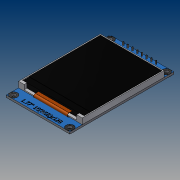
# Autodesk Inventor part: 1e77-TFT-160x128
Saved by Autodesk Inventor 2022.3 (Build 263350000, 350)
## iProperties
Created: 2022-05-13
Part Number: 1e77-TFT-160x128
Material: Generico
Document SubType Name: Modeling
Designer: Bat
Density: 1 g/cm^3
Appearance: Default
Peso: =<MASS>
Author: Bat
Autodesk Inventor part; units mm, degrees
(part 1 of 2)
ref_plane "YZ Plane" through (0, 0, 0) normal (1, 0, 0) x (0, 1, 0)
ref_plane "XZ Plane" through (0, 0, 0) normal (0, 1, 0) x (-1, 0, 0)
ref_plane "XY Plane" through (0, 0, 0) normal (0, 0, 1) x (1, 0, 0)
sketch "Schizzo1" plane through (0, 0, 0) normal (0, 0, 1) x (1, 0, 0)
  line L0 (-17, 27.75) -> (17, 27.75)
  line L1 (17, 27.75) -> (17, -27.75)
  line L2 (17, -27.75) -> (-17, -27.75)
  line L3 (-17, -27.75) -> (-17, 27.75)
  line L4 (-17, 27.75) -> (17, -27.75) construction
  line L5 (17, 27.75) -> (-17, -27.75) construction
  point P0 (0, 0)
  dimension "d0" = 34
  dimension "d1" = 55.5
  constraints: 12 end point, 2 midpoint, 2 parallel, 1 horizontal, 1 perpendicular
  measures "d0" distance of L1.end L2.end
  measures "d1" distance of L0.end L1.end
extrude "Estrusione1" add sketch "Schizzo1" along normal mid plane 1.1
sketch "Schizzo2" plane through (0, 0, 0.55) normal (0, 0, 1) x (1, 0, 0)
  line L0 (-15, -25.75) -> (15, -25.75)
  line L1 (15, -25.75) -> (15, 25.75)
  line L2 (15, 25.75) -> (-15, 25.75)
  line L3 (-15, 25.75) -> (-15, -25.75)
  line L4 (-15, -25.75) -> (15, 25.75) construction
  line L5 (15, -25.75) -> (-15, 25.75) construction
  point P0 (0, 0)
  dimension "d4" = 30
  dimension "d5" = 51.5
  constraints: 12 end point, 2 midpoint, 2 parallel, 1 horizontal, 1 perpendicular
  measures "d4" distance of L1.end L2.end
  measures "d5" distance of L0.end L1.end
hole "Foro1" at (-15, 25.75, 0.55) at (15, 25.75, 0.55) at (-15, -25.75, 0.55) at (15, -25.75, 0.55) direction (0, 0, -1) diameter 2.1 end through all
sketch "Schizzo3" plane through (0, 0, 0.55) normal (0, 0, 1) x (1, 0, 0)
  circle A0 centre (-15, 25.75) radius 1.05 projected
  circle A1 centre (-15, 25.75) radius 2
  line L0 (-23.8, 0) -> (23.8, 0) construction
  line L1 (0, 38.85) -> (0, -38.85) construction
  circle A2 centre (15, 25.75) radius 1.05
  circle A3 centre (15, 25.75) radius 2
  circle A4 centre (-15, -25.75) radius 1.05
  circle A5 centre (-15, -25.75) radius 2
  circle A6 centre (15, -25.75) radius 2
  circle A7 centre (15, -25.75) radius 1.05
  point P0 (0, 0)
  dimension "d13" = 4
  constraints: 7 centre point, 6 symmetric about line, 4 coincident, 6 other
  measures "d13" diameter of A1
extrude "Estrusione2" add sketch "Schizzo3" along normal blind 0.05
mirror "Specchio1" about plane through (0, 0, 0) normal (0, 0, 1) of "Estrusione2"
sketch "Schizzo4" plane through (0, 0, 0.55) normal (0, 0, 1) x (1, 0, 0)
  line L0 (-9, 12.35) -> (-3.8, 12.35)
  line L1 (-3.8, 12.35) -> (-3.8, 9.55)
  line L2 (-3.8, 9.55) -> (-9, 9.55)
  line L3 (-9, 9.55) -> (-9, 12.35)
  line L4 (-9, 12.35) -> (-3.8, 9.55) construction
  line L5 (-3.8, 12.35) -> (-9, 9.55) construction
  line L6 (15, 27.75) -> (-15, 27.75) construction
  line L7 (-17, 25.75) -> (-17, -25.75) construction
  line L8 (-9, 9.15) -> (-3.8, 9.15)
  line L9 (-3.8, 9.15) -> (-3.8, 6.35)
  line L10 (-3.8, 6.35) -> (-9, 6.35)
  line L11 (-9, 6.35) -> (-9, 9.15)
  line L12 (-9, 9.15) -> (-3.8, 6.35) construction
  line L13 (-3.8, 9.15) -> (-9, 6.35) construction
  line L14 (-9, 5.95) -> (-3.8, 5.95)
  line L15 (-3.8, 5.95) -> (-3.8, 3.15)
  line L16 (-3.8, 3.15) -> (-9, 3.15)
  line L17 (-9, 3.15) -> (-9, 5.95)
  line L18 (-9, 5.95) -> (-3.8, 3.15) construction
  line L19 (-3.8, 5.95) -> (-9, 3.15) construction
  line L20 (-2, 7.95) -> (3.2, 7.95)
  line L21 (3.2, 7.95) -> (3.2, 10.75)
  line L22 (3.2, 10.75) -> (-2, 10.75)
  line L23 (-2, 10.75) -> (-2, 7.95)
  line L24 (-2, 7.95) -> (3.2, 10.75) construction
  line L25 (3.2, 7.95) -> (-2, 10.75) construction
  line L26 (-2, 7.55) -> (3.2, 7.55)
  line L27 (3.2, 7.55) -> (3.2, 4.75)
  line L28 (3.2, 4.75) -> (-2, 4.75)
  line L29 (-2, 4.75) -> (-2, 7.55)
  line L30 (-2, 7.55) -> (3.2, 4.75) construction
  line L31 (3.2, 7.55) -> (-2, 4.75) construction
  line L32 (6.3, 13.25) -> (11.5, 13.25)
  line L33 (11.5, 13.25) -> (11.5, 10.45)
  line L34 (11.5, 10.45) -> (6.3, 10.45)
  line L35 (6.3, 10.45) -> (6.3, 13.25)
  line L36 (6.3, 13.25) -> (11.5, 10.45) construction
  line L37 (11.5, 13.25) -> (6.3, 10.45) construction
  line L38 (17, -25.75) -> (17, 25.75) construction
  line L39 (-11.7056, 11.7024) -> (-9.3, 11.7024) construction
  line L40 (-9.3, 11.7024) -> (-9.3, 10.1976) construction
  line L41 (-9.3, 10.1976) -> (-11.7056, 10.1976) construction
  line L42 (-11.7056, 10.1976) -> (-11.7056, 11.7024) construction
  line L43 (-11.7056, 8.5024) -> (-9.3, 8.5024) construction
  line L44 (-9.3, 8.5024) -> (-9.3, 6.9976) construction
  line L45 (-9.3, 6.9976) -> (-11.7056, 6.9976) construction
  line L46 (-11.7056, 6.9976) -> (-11.7056, 8.5024) construction
  line L47 (-11.7056, 5.3024) -> (-9.3, 5.3024) construction
  line L48 (-9.3, 5.3024) -> (-9.3, 3.7976) construction
  line L49 (-9.3, 3.7976) -> (-11.7056, 3.7976) construction
  line L50 (-11.7056, 3.7976) -> (-11.7056, 5.3024) construction
  line L51 (3.5, 10.1024) -> (5.9056, 10.1024) construction
  line L52 (5.9056, 10.1024) -> (5.9056, 8.5976) construction
  line L53 (5.9056, 8.5976) -> (3.5, 8.5976) construction
  line L54 (3.5, 8.5976) -> (3.5, 10.1024) construction
  line L55 (3.5, 5.3976) -> (3.5, 6.9024) construction
  line L56 (3.5, 6.9024) -> (5.9056, 6.9024) construction
  line L57 (5.9056, 6.9024) -> (5.9056, 5.3976) construction
  line L58 (5.9056, 5.3976) -> (3.5, 5.3976) construction
  line L59 (11.8, 11.0976) -> (11.8, 12.6024) construction
  line L60 (11.8, 12.6024) -> (14.2056, 12.6024) construction
  line L61 (14.2056, 12.6024) -> (14.2056, 11.0976) construction
  line L62 (14.2056, 11.0976) -> (11.8, 11.0976) construction
  line L63 (6.3, 16.25) -> (9.8, 16.25)
  line L64 (9.8, 16.25) -> (9.8, 14.25)
  line L65 (9.8, 14.25) -> (6.3, 14.25)
  line L66 (6.3, 14.25) -> (6.3, 16.25)
  line L67 (6.3, 16.25) -> (9.8, 14.25) construction
  line L68 (9.8, 16.25) -> (6.3, 14.25) construction
  line L69 (10.1951, 16.4758) -> (10.1951, 17.9806) construction
  line L70 (10.1951, 17.9806) -> (12.6007, 17.9806) construction
  line L71 (12.6007, 17.9806) -> (12.6007, 16.4758) construction
  line L72 (12.6007, 16.4758) -> (10.1951, 16.4758) construction
  line L73 (-1.2, 15.8215) -> (-0.2, 15.8215)
  line L74 (-0.2, 15.8215) -> (-0.2, 13.3215)
  line L75 (-0.2, 13.3215) -> (-1.2, 13.3215)
  line L76 (-1.2, 13.3215) -> (-1.2, 15.8215)
  line L77 (-1.2, 15.8215) -> (-0.2, 13.3215) construction
  line L78 (-0.2, 15.8215) -> (-1.2, 13.3215) construction
  line L79 (0.1593, 15.9667) -> (0.1593, 17.4716) construction
  line L80 (0.1593, 17.4716) -> (2.5649, 17.4716) construction
  line L81 (2.5649, 17.4716) -> (2.5649, 15.9667) construction
  line L82 (2.5649, 15.9667) -> (0.1593, 15.9667) construction
  line L83 (-13.9282, 19.8471) -> (-2.7925, 19.8471) construction
  line L84 (-2.7925, 19.8471) -> (-2.7925, 18.2669) construction
  line L85 (-2.7925, 18.2669) -> (-13.9282, 18.2669) construction
  line L86 (-13.9282, 18.2669) -> (-13.9282, 19.8471) construction
  line L87 (-3.95, 12.2) -> (-8.85, 12.2)
  line L88 (-8.85, 12.2) -> (-8.85, 9.7)
  line L89 (-8.85, 9.7) -> (-3.95, 9.7)
  line L90 (-3.95, 9.7) -> (-3.95, 12.2)
  line L91 (-3.95, 9) -> (-8.85, 9)
  line L92 (-8.85, 9) -> (-8.85, 6.5)
  line L93 (-8.85, 6.5) -> (-3.95, 6.5)
  line L94 (-3.95, 6.5) -> (-3.95, 9)
  line L95 (-3.95, 5.8) -> (-8.85, 5.8)
  line L96 (-8.85, 5.8) -> (-8.85, 3.3)
  line L97 (-8.85, 3.3) -> (-3.95, 3.3)
  line L98 (-3.95, 3.3) -> (-3.95, 5.8)
  line L99 (-1.85, 10.6) -> (3.05, 10.6)
  line L100 (3.05, 10.6) -> (3.05, 8.1)
  line L101 (3.05, 8.1) -> (-1.85, 8.1)
  line L102 (-1.85, 8.1) -> (-1.85, 10.6)
  line L103 (3.05, 7.4) -> (-1.85, 7.4)
  line L104 (-1.85, 7.4) -> (-1.85, 4.9)
  line L105 (-1.85, 4.9) -> (3.05, 4.9)
  line L106 (3.05, 4.9) -> (3.05, 7.4)
  line L107 (11.35, 13.1) -> (6.45, 13.1)
  line L108 (6.45, 13.1) -> (6.45, 10.6)
  line L109 (6.45, 10.6) -> (11.35, 10.6)
  line L110 (11.35, 10.6) -> (11.35, 13.1)
  line L111 (9.65, 16.1) -> (6.45, 16.1)
  line L112 (6.45, 16.1) -> (6.45, 14.4)
  line L113 (6.45, 14.4) -> (9.65, 14.4)
  line L114 (9.65, 14.4) -> (9.65, 16.1)
  line L115 (-0.35, 15.6715) -> (-1.05, 15.6715)
  line L116 (-1.05, 15.6715) -> (-1.05, 13.4715)
  line L117 (-1.05, 13.4715) -> (-0.35, 13.4715)
  line L118 (-0.35, 13.4715) -> (-0.35, 15.6715)
  line L119 (-10.3928, 10.1976) -> (-10.6517, 10.1976)
  line L120 (-10.6517, 10.1976) -> (-11.1258, 10.7944)
  line L121 (-11.1258, 10.7944) -> (-11.3543, 10.7944)
  line L122 (-11.3543, 10.7944) -> (-11.3543, 10.1976)
  line L123 (-11.3543, 10.1976) -> (-11.5536, 10.1976)
  line L124 (-11.5536, 10.1976) -> (-11.5536, 11.6976)
  line L125 (-11.5536, 11.6976) -> (-11.1671, 11.6976)
  spline S0 degree 2 poles (-11.1671, 11.6976) (-11.0382, 11.6976) (-10.8644, 11.6696) (-10.7854, 11.6186) knots 0 0 0 1 2 2 2
  spline S1 degree 2 poles (-10.7854, 11.6186) (-10.7064, 11.5675) (-10.6152, 11.4083) (-10.6152, 11.2904) knots 0 0 0 1 2 2 2
  spline S2 degree 2 poles (-10.6152, 11.2904) (-10.6152, 11.1263) (-10.783, 10.9038) (-10.9264, 10.8503) knots 0 0 0 1 2 2 2
  line L126 (-10.9264, 10.8503) -> (-10.3928, 10.1976)
  spline S3 degree 2 poles (-10.8231, 11.2746) (-10.8231, 11.3402) (-10.8693, 11.4411) (-10.9179, 11.4739) knots 0 0 0 1 2 2 2
  spline S4 degree 2 poles (-10.9179, 11.4739) (-10.9605, 11.5019) (-11.0735, 11.525) (-11.1562, 11.525) knots 0 0 0 1 2 2 2
  line L127 (-11.1562, 11.525) -> (-11.3543, 11.525)
  line L128 (-11.3543, 11.525) -> (-11.3543, 10.9609)
  line L129 (-11.3543, 10.9609) -> (-11.1793, 10.9609)
  spline S5 degree 2 poles (-11.1793, 10.9609) (-11.0929, 10.9609) (-10.9556, 10.9913) (-10.9082, 11.0387) knots 0 0 0 1 2 2 2
  spline S6 degree 2 poles (-10.9082, 11.0387) (-10.8644, 11.0801) (-10.8231, 11.1968) (-10.8231, 11.2746) knots 0 0 0 1 2 2 2
  line L130 (-9.4665, 10.1976) -> (-10.1983, 10.1976)
  line L131 (-10.1983, 10.1976) -> (-10.1983, 10.3507)
  line L132 (-10.1983, 10.3507) -> (-9.926, 10.3507)
  line L133 (-9.926, 10.3507) -> (-9.926, 11.356)
  line L134 (-9.926, 11.356) -> (-10.1983, 11.356)
  line L135 (-10.1983, 11.356) -> (-10.1983, 11.4934)
  spline S7 degree 2 poles (-10.1983, 11.4934) (-10.0439, 11.4934) (-9.8981, 11.5809) (-9.8883, 11.7024) knots 0 0 0 1 2 2 2
  line L136 (-9.8883, 11.7024) -> (-9.7327, 11.7024)
  line L137 (-9.7327, 11.7024) -> (-9.7327, 10.3507)
  line L138 (-9.7327, 10.3507) -> (-9.4665, 10.3507)
  line L139 (-9.4665, 10.3507) -> (-9.4665, 10.1976)
  spline S8 degree 2 poles (0.7, 16.1045) (0.594, 16.1045) (0.4364, 16.16) (0.381, 16.2154) knots 0 0 0 1 2 2 2
  spline S9 degree 2 poles (0.381, 16.2154) (0.3178, 16.2776) (0.2663, 16.4527) (0.2663, 16.581) knots 0 0 0 1 2 2 2
  line L140 (0.2663, 16.581) -> (0.2663, 17.3298)
  line L141 (0.2663, 17.3298) -> (0.4257, 17.3298)
  line L142 (0.4257, 17.3298) -> (0.4257, 16.581)
  spline S10 degree 2 poles (0.4257, 16.581) (0.4257, 16.4974) (0.4471, 16.3846) (0.4773, 16.3389) knots 0 0 0 1 2 2 2
  spline S11 degree 2 poles (0.4773, 16.3389) (0.5094, 16.2903) (0.6202, 16.2407) (0.7, 16.2407) knots 0 0 0 1 2 2 2
  spline S12 degree 2 poles (0.7, 16.2407) (0.7748, 16.2407) (0.8915, 16.2903) (0.9236, 16.3389) knots 0 0 0 1 2 2 2
  spline S13 degree 2 poles (0.9236, 16.3389) (0.9538, 16.3846) (0.9752, 16.4964) (0.9752, 16.5772) knots 0 0 0 1 2 2 2
  line L143 (0.9752, 16.5772) -> (0.9752, 17.3298)
  line L144 (0.9752, 17.3298) -> (1.1346, 17.3298)
  line L145 (1.1346, 17.3298) -> (1.1346, 16.581)
  spline S14 degree 2 poles (1.1346, 16.581) (1.1346, 16.4556) (1.0841, 16.2767) (1.0199, 16.2154) knots 0 0 0 1 2 2 2
  spline S15 degree 2 poles (1.0199, 16.2154) (0.9625, 16.159) (0.8108, 16.1045) (0.7, 16.1045) knots 0 0 0 1 2 2 2
  line L146 (2.0089, 16.1298) -> (1.4235, 16.1298)
  line L147 (1.4235, 16.1298) -> (1.4235, 16.2524)
  line L148 (1.4235, 16.2524) -> (1.6413, 16.2524)
  line L149 (1.6413, 16.2524) -> (1.6413, 17.0566)
  line L150 (1.6413, 17.0566) -> (1.4235, 17.0566)
  line L151 (1.4235, 17.0566) -> (1.4235, 17.1665)
  spline S16 degree 2 poles (1.4235, 17.1665) (1.547, 17.1665) (1.6637, 17.2365) (1.6714, 17.3337) knots 0 0 0 1 2 2 2
  line L152 (1.6714, 17.3337) -> (1.7959, 17.3337)
  line L153 (1.7959, 17.3337) -> (1.7959, 16.2524)
  line L154 (1.7959, 16.2524) -> (2.0089, 16.2524)
  line L155 (2.0089, 16.2524) -> (2.0089, 16.1298)
  line L156 (-12.794, 17.1939) -> (-13.6585, 17.1939)
  line L157 (-13.6585, 17.1939) -> (-13.6585, 17.4533)
  line L158 (-13.6585, 17.4533) -> (-13.3374, 17.4533)
  line L159 (-13.3374, 17.4533) -> (-13.3374, 19.1555)
  line L160 (-13.3374, 19.1555) -> (-13.6585, 19.1555)
  line L161 (-13.6585, 19.1555) -> (-13.6585, 19.3881)
  spline S17 degree 2 poles (-13.6585, 19.3881) (-13.4774, 19.3881) (-13.3045, 19.5363) (-13.2942, 19.7422) knots 0 0 0 1 2 2 2
  line L162 (-13.2942, 19.7422) -> (-13.109, 19.7422)
  line L163 (-13.109, 19.7422) -> (-13.109, 17.4533)
  line L164 (-13.109, 17.4533) -> (-12.794, 17.4533)
  line L165 (-12.794, 17.4533) -> (-12.794, 17.1939)
  line L166 (-12.0839, 17.1939) -> (-12.368, 17.1939)
  line L167 (-12.368, 17.1939) -> (-12.368, 17.6797)
  line L168 (-12.368, 17.6797) -> (-12.0839, 17.6797)
  line L169 (-12.0839, 17.6797) -> (-12.0839, 17.1939)
  line L170 (-10.6122, 19.3531) -> (-11.38, 17.1939)
  line L171 (-11.38, 17.1939) -> (-11.6331, 17.1939)
  line L172 (-11.6331, 17.1939) -> (-10.8221, 19.4355)
  line L173 (-10.8221, 19.4355) -> (-11.7381, 19.4355)
  line L174 (-11.7381, 19.4355) -> (-11.7381, 19.7339)
  line L175 (-11.7381, 19.7339) -> (-10.6122, 19.7339)
  line L176 (-10.6122, 19.7339) -> (-10.6122, 19.3531)
  line L177 (-9.2784, 19.3531) -> (-10.0462, 17.1939)
  line L178 (-10.0462, 17.1939) -> (-10.2993, 17.1939)
  line L179 (-10.2993, 17.1939) -> (-9.4883, 19.4355)
  line L180 (-9.4883, 19.4355) -> (-10.4043, 19.4355)
  line L181 (-10.4043, 19.4355) -> (-10.4043, 19.7339)
  line L182 (-10.4043, 19.7339) -> (-9.2784, 19.7339)
  line L183 (-9.2784, 19.7339) -> (-9.2784, 19.3531)
  line L184 (-8.3439, 19.8471) -> (-8.3954, 18.8591)
  line L185 (-8.3954, 18.8591) -> (-8.5518, 18.8591)
  line L186 (-8.5518, 18.8591) -> (-8.6032, 19.8471)
  line L187 (-8.6032, 19.8471) -> (-8.3439, 19.8471)
  line L188 (-8.7926, 19.8471) -> (-8.8441, 18.8591)
  line L189 (-8.8441, 18.8591) -> (-9.0005, 18.8591)
  line L190 (-9.0005, 18.8591) -> (-9.052, 19.8471)
  line L191 (-9.052, 19.8471) -> (-8.7926, 19.8471)
  line L192 (-6.8495, 17.1939) -> (-6.8495, 19.4334)
  line L193 (-6.8495, 19.4334) -> (-7.4465, 19.4334)
  line L194 (-7.4465, 19.4334) -> (-7.4465, 19.7339)
  line L195 (-7.4465, 19.7339) -> (-6.0159, 19.7339)
  line L196 (-6.0159, 19.7339) -> (-6.0159, 19.4334)
  line L197 (-6.0159, 19.4334) -> (-6.6128, 19.4334)
  line L198 (-6.6128, 19.4334) -> (-6.6128, 17.1939)
  line L199 (-6.6128, 17.1939) -> (-6.8495, 17.1939)
  line L200 (-4.7768, 19.4334) -> (-5.6022, 19.4334)
  line L201 (-5.6022, 19.4334) -> (-5.6022, 18.7171)
  line L202 (-5.6022, 18.7171) -> (-4.8118, 18.7171)
  line L203 (-4.8118, 18.7171) -> (-4.8118, 18.4166)
  line L204 (-4.8118, 18.4166) -> (-5.6022, 18.4166)
  line L205 (-5.6022, 18.4166) -> (-5.6022, 17.1939)
  line L206 (-5.6022, 17.1939) -> (-5.8389, 17.1939)
  line L207 (-5.8389, 17.1939) -> (-5.8389, 19.7339)
  line L208 (-5.8389, 19.7339) -> (-4.7768, 19.7339)
  line L209 (-4.7768, 19.7339) -> (-4.7768, 19.4334)
  line L210 (-4.149, 17.1939) -> (-4.149, 19.4334)
  line L211 (-4.149, 19.4334) -> (-4.7459, 19.4334)
  line L212 (-4.7459, 19.4334) -> (-4.7459, 19.7339)
  line L213 (-4.7459, 19.7339) -> (-3.3154, 19.7339)
  line L214 (-3.3154, 19.7339) -> (-3.3154, 19.4334)
  line L215 (-3.3154, 19.4334) -> (-3.9123, 19.4334)
  line L216 (-3.9123, 19.4334) -> (-3.9123, 17.1939)
  line L217 (-3.9123, 17.1939) -> (-4.149, 17.1939)
  line L218 (-10.3928, 7) -> (-10.6517, 7)
  line L219 (-10.6517, 7) -> (-11.1258, 7.5968)
  line L220 (-11.1258, 7.5968) -> (-11.3543, 7.5968)
  line L221 (-11.3543, 7.5968) -> (-11.3543, 7)
  line L222 (-11.3543, 7) -> (-11.5536, 7)
  line L223 (-11.5536, 7) -> (-11.5536, 8.5)
  line L224 (-11.5536, 8.5) -> (-11.1671, 8.5)
  spline S18 degree 2 poles (-11.1671, 8.5) (-11.0382, 8.5) (-10.8644, 8.472) (-10.7854, 8.421) knots 0 0 0 1 2 2 2
  spline S19 degree 2 poles (-10.7854, 8.421) (-10.7064, 8.3699) (-10.6152, 8.2107) (-10.6152, 8.0928) knots 0 0 0 1 2 2 2
  spline S20 degree 2 poles (-10.6152, 8.0928) (-10.6152, 7.9287) (-10.783, 7.7062) (-10.9264, 7.6528) knots 0 0 0 1 2 2 2
  line L225 (-10.9264, 7.6528) -> (-10.3928, 7)
  spline S21 degree 2 poles (-10.8231, 8.077) (-10.8231, 8.1426) (-10.8693, 8.2435) (-10.9179, 8.2763) knots 0 0 0 1 2 2 2
  spline S22 degree 2 poles (-10.9179, 8.2763) (-10.9605, 8.3043) (-11.0735, 8.3274) (-11.1562, 8.3274) knots 0 0 0 1 2 2 2
  line L226 (-11.1562, 8.3274) -> (-11.3543, 8.3274)
  line L227 (-11.3543, 8.3274) -> (-11.3543, 7.7634)
  line L228 (-11.3543, 7.7634) -> (-11.1793, 7.7634)
  spline S23 degree 2 poles (-11.1793, 7.7634) (-11.0929, 7.7634) (-10.9556, 7.7938) (-10.9082, 7.8412) knots 0 0 0 1 2 2 2
  spline S24 degree 2 poles (-10.9082, 7.8412) (-10.8644, 7.8825) (-10.8231, 7.9992) (-10.8231, 8.077) knots 0 0 0 1 2 2 2
  spline S25 degree 2 poles (-9.9114, 8.3578) (-9.9661, 8.3578) (-10.0743, 8.331) (-10.1266, 8.3104) knots 0 0 0 1 2 2 2
  spline S26 degree 2 poles (-10.1266, 8.3104) (-10.1752, 8.2897) (-10.2469, 8.2459) (-10.2749, 8.2265) knots 0 0 0 1 2 2 2
  line L229 (-10.2749, 8.2265) -> (-10.287, 8.2265)
  line L230 (-10.287, 8.2265) -> (-10.287, 8.4392)
  spline S27 degree 2 poles (-10.287, 8.4392) (-10.2214, 8.4745) (-9.9965, 8.5316) (-9.8956, 8.5316) knots 0 0 0 1 2 2 2
  spline S28 degree 2 poles (-9.8956, 8.5316) (-9.7935, 8.5316) (-9.6416, 8.4903) (-9.5796, 8.4465) knots 0 0 0 1 2 2 2
  spline S29 degree 2 poles (-9.5796, 8.4465) (-9.5139, 8.3991) (-9.4459, 8.2618) (-9.4459, 8.1694) knots 0 0 0 1 2 2 2
  spline S30 degree 2 poles (-9.4459, 8.1694) (-9.4459, 8.0454) (-9.6088, 7.8582) (-9.723, 7.8339) knots 0 0 0 1 2 2 2
  line L231 (-9.723, 7.8339) -> (-9.723, 7.8193)
  spline S31 degree 2 poles (-9.723, 7.8193) (-9.6756, 7.8096) (-9.5674, 7.7658) (-9.5212, 7.722) knots 0 0 0 1 2 2 2
  spline S32 degree 2 poles (-9.5212, 7.722) (-9.475, 7.6795) (-9.4167, 7.5434) (-9.4167, 7.4449) knots 0 0 0 1 2 2 2
  spline S33 degree 2 poles (-9.4167, 7.4449) (-9.4167, 7.344) (-9.486, 7.1726) (-9.5492, 7.107) knots 0 0 0 1 2 2 2
  spline S34 degree 2 poles (-9.5492, 7.107) (-9.6148, 7.0389) (-9.8008, 6.9684) (-9.9187, 6.9684) knots 0 0 0 1 2 2 2
  spline S35 degree 2 poles (-9.9187, 6.9684) (-10.0318, 6.9684) (-10.253, 7.0231) (-10.3284, 7.0608) knots 0 0 0 1 2 2 2
  line L232 (-10.3284, 7.0608) -> (-10.3284, 7.2735)
  line L233 (-10.3284, 7.2735) -> (-10.3138, 7.2735)
  spline S36 degree 2 poles (-10.3138, 7.2735) (-10.2506, 7.2273) (-10.0366, 7.1422) (-9.9309, 7.1422) knots 0 0 0 1 2 2 2
  spline S37 degree 2 poles (-9.9309, 7.1422) (-9.8689, 7.1422) (-9.7449, 7.1811) (-9.7036, 7.2261) knots 0 0 0 1 2 2 2
  spline S38 degree 2 poles (-9.7036, 7.2261) (-9.6635, 7.2711) (-9.6209, 7.378) (-9.6209, 7.4595) knots 0 0 0 1 2 2 2
  spline S39 degree 2 poles (-9.6209, 7.4595) (-9.6209, 7.5409) (-9.6683, 7.6467) (-9.7109, 7.6771) knots 0 0 0 1 2 2 2
  spline S40 degree 2 poles (-9.7109, 7.6771) (-9.7534, 7.7075) (-9.8689, 7.7306) (-9.937, 7.7306) knots 0 0 0 1 2 2 2
  line L234 (-9.937, 7.7306) -> (-10.022, 7.7306)
  line L235 (-10.022, 7.7306) -> (-10.022, 7.8971)
  line L236 (-10.022, 7.8971) -> (-9.9552, 7.8971)
  spline S41 degree 2 poles (-9.9552, 7.8971) (-9.8203, 7.8971) (-9.6501, 8.0259) (-9.6501, 8.1487) knots 0 0 0 1 2 2 2
  spline S42 degree 2 poles (-9.6501, 8.1487) (-9.6501, 8.2058) (-9.6938, 8.2873) (-9.7291, 8.3116) knots 0 0 0 1 2 2 2
  spline S43 degree 2 poles (-9.7291, 8.3116) (-9.7668, 8.3371) (-9.8592, 8.3578) (-9.9114, 8.3578) knots 0 0 0 1 2 2 2
  spline S44 degree 2 poles (-10.9264, 3.7733) (-11.0723, 3.7733) (-11.319, 3.8717) (-11.409, 3.9702) knots 0 0 0 1 2 2 2
  spline S45 degree 2 poles (-11.409, 3.9702) (-11.4989, 4.0674) (-11.5974, 4.3592) (-11.5974, 4.5488) knots 0 0 0 1 2 2 2
  spline S46 degree 2 poles (-11.5974, 4.5488) (-11.5974, 4.7372) (-11.5014, 5.0168) (-11.4102, 5.1201) knots 0 0 0 1 2 2 2
  spline S47 degree 2 poles (-11.4102, 5.1201) (-11.3203, 5.221) (-11.0747, 5.3267) (-10.9228, 5.3267) knots 0 0 0 1 2 2 2
  spline S48 degree 2 poles (-10.9228, 5.3267) (-10.8474, 5.3267) (-10.7149, 5.3049) (-10.659, 5.2878) knots 0 0 0 1 2 2 2
  spline S49 degree 2 poles (-10.659, 5.2878) (-10.6104, 5.272) (-10.5095, 5.2271) (-10.4596, 5.2003) knots 0 0 0 1 2 2 2
  line L237 (-10.4596, 5.2003) -> (-10.4596, 4.9596)
  line L238 (-10.4596, 4.9596) -> (-10.4754, 4.9596)
  spline S50 degree 2 poles (-10.4754, 4.9596) (-10.5022, 4.984) (-10.5848, 5.052) (-10.6444, 5.0848) knots 0 0 0 1 2 2 2
  spline S51 degree 2 poles (-10.6444, 5.0848) (-10.7015, 5.1165) (-10.8365, 5.1566) (-10.924, 5.1566) knots 0 0 0 1 2 2 2
  spline S52 degree 2 poles (-10.924, 5.1566) (-11.02, 5.1566) (-11.1914, 5.0776) (-11.2558, 5.0022) knots 0 0 0 1 2 2 2
  spline S53 degree 2 poles (-11.2558, 5.0022) (-11.319, 4.9256) (-11.3895, 4.6934) (-11.3895, 4.5488) knots 0 0 0 1 2 2 2
  spline S54 degree 2 poles (-11.3895, 4.5488) (-11.3895, 4.3944) (-11.3154, 4.172) (-11.251, 4.0954) knots 0 0 0 1 2 2 2
  spline S55 degree 2 poles (-11.251, 4.0954) (-11.1878, 4.0212) (-11.0188, 3.9459) (-10.924, 3.9459) knots 0 0 0 1 2 2 2
  spline S56 degree 2 poles (-10.924, 3.9459) (-10.8377, 3.9459) (-10.6906, 3.9884) (-10.6335, 4.02) knots 0 0 0 1 2 2 2
  spline S57 degree 2 poles (-10.6335, 4.02) (-10.5788, 4.0516) (-10.4973, 4.1173) (-10.4742, 4.1404) knots 0 0 0 1 2 2 2
  line L239 (-10.4742, 4.1404) -> (-10.4596, 4.1404)
  line L240 (-10.4596, 4.1404) -> (-10.4596, 3.9021)
  spline S58 degree 2 poles (-10.4596, 3.9021) (-10.5095, 3.879) (-10.597, 3.8365) (-10.659, 3.817) knots 0 0 0 1 2 2 2
  spline S59 degree 2 poles (-10.659, 3.817) (-10.7246, 3.7951) (-10.8365, 3.7733) (-10.9264, 3.7733) knots 0 0 0 1 2 2 2
  spline S60 degree 2 poles (-9.9114, 5.1578) (-9.9661, 5.1578) (-10.0743, 5.131) (-10.1266, 5.1104) knots 0 0 0 1 2 2 2
  spline S61 degree 2 poles (-10.1266, 5.1104) (-10.1752, 5.0897) (-10.2469, 5.0459) (-10.2749, 5.0265) knots 0 0 0 1 2 2 2
  line L241 (-10.2749, 5.0265) -> (-10.287, 5.0265)
  line L242 (-10.287, 5.0265) -> (-10.287, 5.2392)
  spline S62 degree 2 poles (-10.287, 5.2392) (-10.2214, 5.2745) (-9.9965, 5.3316) (-9.8956, 5.3316) knots 0 0 0 1 2 2 2
  spline S63 degree 2 poles (-9.8956, 5.3316) (-9.7935, 5.3316) (-9.6416, 5.2903) (-9.5796, 5.2465) knots 0 0 0 1 2 2 2
  spline S64 degree 2 poles (-9.5796, 5.2465) (-9.5139, 5.1991) (-9.4459, 5.0618) (-9.4459, 4.9694) knots 0 0 0 1 2 2 2
  spline S65 degree 2 poles (-9.4459, 4.9694) (-9.4459, 4.8454) (-9.6088, 4.6582) (-9.723, 4.6339) knots 0 0 0 1 2 2 2
  line L243 (-9.723, 4.6339) -> (-9.723, 4.6193)
  spline S66 degree 2 poles (-9.723, 4.6193) (-9.6756, 4.6096) (-9.5674, 4.5658) (-9.5212, 4.522) knots 0 0 0 1 2 2 2
  spline S67 degree 2 poles (-9.5212, 4.522) (-9.475, 4.4795) (-9.4167, 4.3434) (-9.4167, 4.2449) knots 0 0 0 1 2 2 2
  spline S68 degree 2 poles (-9.4167, 4.2449) (-9.4167, 4.144) (-9.486, 3.9726) (-9.5492, 3.907) knots 0 0 0 1 2 2 2
  spline S69 degree 2 poles (-9.5492, 3.907) (-9.6148, 3.8389) (-9.8008, 3.7684) (-9.9187, 3.7684) knots 0 0 0 1 2 2 2
  spline S70 degree 2 poles (-9.9187, 3.7684) (-10.0318, 3.7684) (-10.253, 3.8231) (-10.3284, 3.8608) knots 0 0 0 1 2 2 2
  line L244 (-10.3284, 3.8608) -> (-10.3284, 4.0735)
  line L245 (-10.3284, 4.0735) -> (-10.3138, 4.0735)
  spline S71 degree 2 poles (-10.3138, 4.0735) (-10.2506, 4.0273) (-10.0366, 3.9422) (-9.9309, 3.9422) knots 0 0 0 1 2 2 2
  spline S72 degree 2 poles (-9.9309, 3.9422) (-9.8689, 3.9422) (-9.7449, 3.9811) (-9.7036, 4.0261) knots 0 0 0 1 2 2 2
  spline S73 degree 2 poles (-9.7036, 4.0261) (-9.6635, 4.0711) (-9.6209, 4.178) (-9.6209, 4.2595) knots 0 0 0 1 2 2 2
  spline S74 degree 2 poles (-9.6209, 4.2595) (-9.6209, 4.3409) (-9.6683, 4.4467) (-9.7109, 4.4771) knots 0 0 0 1 2 2 2
  spline S75 degree 2 poles (-9.7109, 4.4771) (-9.7534, 4.5075) (-9.8689, 4.5306) (-9.937, 4.5306) knots 0 0 0 1 2 2 2
  line L246 (-9.937, 4.5306) -> (-10.022, 4.5306)
  line L247 (-10.022, 4.5306) -> (-10.022, 4.6971)
  line L248 (-10.022, 4.6971) -> (-9.9552, 4.6971)
  spline S76 degree 2 poles (-9.9552, 4.6971) (-9.8203, 4.6971) (-9.6501, 4.8259) (-9.6501, 4.9487) knots 0 0 0 1 2 2 2
  spline S77 degree 2 poles (-9.6501, 4.9487) (-9.6501, 5.0058) (-9.6938, 5.0873) (-9.7291, 5.1116) knots 0 0 0 1 2 2 2
  spline S78 degree 2 poles (-9.7291, 5.1116) (-9.7668, 5.1371) (-9.8592, 5.1578) (-9.9114, 5.1578) knots 0 0 0 1 2 2 2
  spline S79 degree 2 poles (4.2378, 5.3708) (4.092, 5.3708) (3.8452, 5.4693) (3.7553, 5.5677) knots 0 0 0 1 2 2 2
  spline S80 degree 2 poles (3.7553, 5.5677) (3.6653, 5.665) (3.5669, 5.9567) (3.5669, 6.1464) knots 0 0 0 1 2 2 2
  spline S81 degree 2 poles (3.5669, 6.1464) (3.5669, 6.3348) (3.6629, 6.6143) (3.7541, 6.7177) knots 0 0 0 1 2 2 2
  spline S82 degree 2 poles (3.7541, 6.7177) (3.844, 6.8186) (4.0895, 6.9243) (4.2415, 6.9243) knots 0 0 0 1 2 2 2
  spline S83 degree 2 poles (4.2415, 6.9243) (4.3169, 6.9243) (4.4494, 6.9024) (4.5053, 6.8854) knots 0 0 0 1 2 2 2
  spline S84 degree 2 poles (4.5053, 6.8854) (4.5539, 6.8696) (4.6548, 6.8246) (4.7046, 6.7979) knots 0 0 0 1 2 2 2
  line L249 (4.7046, 6.7979) -> (4.7046, 6.5572)
  line L250 (4.7046, 6.5572) -> (4.6888, 6.5572)
  spline S85 degree 2 poles (4.6888, 6.5572) (4.6621, 6.5815) (4.5794, 6.6496) (4.5199, 6.6824) knots 0 0 0 1 2 2 2
  spline S86 degree 2 poles (4.5199, 6.6824) (4.4627, 6.714) (4.3278, 6.7541) (4.2403, 6.7541) knots 0 0 0 1 2 2 2
  spline S87 degree 2 poles (4.2403, 6.7541) (4.1442, 6.7541) (3.9729, 6.6751) (3.9084, 6.5998) knots 0 0 0 1 2 2 2
  spline S88 degree 2 poles (3.9084, 6.5998) (3.8452, 6.5232) (3.7747, 6.291) (3.7747, 6.1464) knots 0 0 0 1 2 2 2
  spline S89 degree 2 poles (3.7747, 6.1464) (3.7747, 5.992) (3.8489, 5.7695) (3.9133, 5.6929) knots 0 0 0 1 2 2 2
  spline S90 degree 2 poles (3.9133, 5.6929) (3.9765, 5.6188) (4.1455, 5.5434) (4.2403, 5.5434) knots 0 0 0 1 2 2 2
  spline S91 degree 2 poles (4.2403, 5.5434) (4.3266, 5.5434) (4.4737, 5.586) (4.5308, 5.6176) knots 0 0 0 1 2 2 2
  spline S92 degree 2 poles (4.5308, 5.6176) (4.5855, 5.6492) (4.6669, 5.7148) (4.69, 5.7379) knots 0 0 0 1 2 2 2
  line L251 (4.69, 5.7379) -> (4.7046, 5.7379)
  line L252 (4.7046, 5.7379) -> (4.7046, 5.4997)
  spline S93 degree 2 poles (4.7046, 5.4997) (4.6548, 5.4766) (4.5673, 5.434) (4.5053, 5.4146) knots 0 0 0 1 2 2 2
  spline S94 degree 2 poles (4.5053, 5.4146) (4.4396, 5.3927) (4.3278, 5.3708) (4.2378, 5.3708) knots 0 0 0 1 2 2 2
  line L253 (5.7731, 5.3976) -> (4.8481, 5.3976)
  line L254 (4.8481, 5.3976) -> (4.8481, 5.6103)
  spline S95 degree 2 poles (4.8481, 5.6103) (4.9477, 5.7039) (5.1252, 5.8777) (5.2103, 5.9713) knots 0 0 0 1 2 2 2
  spline S96 degree 2 poles (5.2103, 5.9713) (5.3817, 6.1597) (5.5069, 6.3858) (5.5069, 6.5062) knots 0 0 0 1 2 2 2
  spline S97 degree 2 poles (5.5069, 6.5062) (5.5069, 6.5694) (5.468, 6.6642) (5.4327, 6.6946) knots 0 0 0 1 2 2 2
  spline S98 degree 2 poles (5.4327, 6.6946) (5.3975, 6.725) (5.3051, 6.7553) (5.2492, 6.7553) knots 0 0 0 1 2 2 2
  spline S99 degree 2 poles (5.2492, 6.7553) (5.1957, 6.7553) (5.0863, 6.7286) (5.0365, 6.7079) knots 0 0 0 1 2 2 2
  spline S100 degree 2 poles (5.0365, 6.7079) (4.9939, 6.6909) (4.9149, 6.6423) (4.8906, 6.6253) knots 0 0 0 1 2 2 2
  line L255 (4.8906, 6.6253) -> (4.8797, 6.6253)
  line L256 (4.8797, 6.6253) -> (4.8797, 6.8392)
  spline S101 degree 2 poles (4.8797, 6.8392) (4.9417, 6.8696) (5.1641, 6.9292) (5.2638, 6.9292) knots 0 0 0 1 2 2 2
  spline S102 degree 2 poles (5.2638, 6.9292) (5.4741, 6.9292) (5.7111, 6.7067) (5.7111, 6.5171) knots 0 0 0 1 2 2 2
  spline S103 degree 2 poles (5.7111, 6.5171) (5.7111, 6.4284) (5.6698, 6.2801) (5.6333, 6.2169) knots 0 0 0 1 2 2 2
  spline S104 degree 2 poles (5.6333, 6.2169) (5.5968, 6.1512) (5.4911, 6.0224) (5.4327, 5.9604) knots 0 0 0 1 2 2 2
  spline S105 degree 2 poles (5.4327, 5.9604) (5.3379, 5.8571) (5.1058, 5.6358) (5.0365, 5.5714) knots 0 0 0 1 2 2 2
  line L257 (5.0365, 5.5714) -> (5.7731, 5.5714)
  line L258 (5.7731, 5.5714) -> (5.7731, 5.3976)
  line L259 (4.8128, 8.5842) -> (4.5539, 8.5842)
  line L260 (4.5539, 8.5842) -> (4.0798, 9.181)
  line L261 (4.0798, 9.181) -> (3.8513, 9.181)
  line L262 (3.8513, 9.181) -> (3.8513, 8.5842)
  line L263 (3.8513, 8.5842) -> (3.6519, 8.5842)
  line L264 (3.6519, 8.5842) -> (3.6519, 10.0842)
  line L265 (3.6519, 10.0842) -> (4.0385, 10.0842)
  spline S106 degree 2 poles (4.0385, 10.0842) (4.1673, 10.0842) (4.3412, 10.0562) (4.4202, 10.0052) knots 0 0 0 1 2 2 2
  spline S107 degree 2 poles (4.4202, 10.0052) (4.4992, 9.9541) (4.5904, 9.7949) (4.5904, 9.677) knots 0 0 0 1 2 2 2
  spline S108 degree 2 poles (4.5904, 9.677) (4.5904, 9.5129) (4.4226, 9.2904) (4.2792, 9.237) knots 0 0 0 1 2 2 2
  line L266 (4.2792, 9.237) -> (4.8128, 8.5842)
  spline S109 degree 2 poles (4.3825, 9.6612) (4.3825, 9.7268) (4.3363, 9.8277) (4.2877, 9.8605) knots 0 0 0 1 2 2 2
  spline S110 degree 2 poles (4.2877, 9.8605) (4.2451, 9.8885) (4.1321, 9.9116) (4.0494, 9.9116) knots 0 0 0 1 2 2 2
  line L267 (4.0494, 9.9116) -> (3.8513, 9.9116)
  line L268 (3.8513, 9.9116) -> (3.8513, 9.3476)
  line L269 (3.8513, 9.3476) -> (4.0263, 9.3476)
  spline S111 degree 2 poles (4.0263, 9.3476) (4.1126, 9.3476) (4.25, 9.378) (4.2974, 9.4254) knots 0 0 0 1 2 2 2
  spline S112 degree 2 poles (4.2974, 9.4254) (4.3412, 9.4667) (4.3825, 9.5834) (4.3825, 9.6612) knots 0 0 0 1 2 2 2
  line L270 (5.8144, 8.5842) -> (4.8894, 8.5842)
  line L271 (4.8894, 8.5842) -> (4.8894, 8.7969)
  spline S113 degree 2 poles (4.8894, 8.7969) (4.9891, 8.8905) (5.1665, 9.0643) (5.2516, 9.1579) knots 0 0 0 1 2 2 2
  spline S114 degree 2 poles (5.2516, 9.1579) (5.423, 9.3464) (5.5482, 9.5724) (5.5482, 9.6928) knots 0 0 0 1 2 2 2
  spline S115 degree 2 poles (5.5482, 9.6928) (5.5482, 9.756) (5.5093, 9.8508) (5.4741, 9.8812) knots 0 0 0 1 2 2 2
  spline S116 degree 2 poles (5.4741, 9.8812) (5.4388, 9.9116) (5.3464, 9.942) (5.2905, 9.942) knots 0 0 0 1 2 2 2
  spline S117 degree 2 poles (5.2905, 9.942) (5.237, 9.942) (5.1276, 9.9152) (5.0778, 9.8946) knots 0 0 0 1 2 2 2
  spline S118 degree 2 poles (5.0778, 9.8946) (5.0353, 9.8776) (4.9562, 9.8289) (4.9319, 9.8119) knots 0 0 0 1 2 2 2
  line L272 (4.9319, 9.8119) -> (4.921, 9.8119)
  line L273 (4.921, 9.8119) -> (4.921, 10.0259)
  spline S119 degree 2 poles (4.921, 10.0259) (4.983, 10.0562) (5.2054, 10.1158) (5.3051, 10.1158) knots 0 0 0 1 2 2 2
  spline S120 degree 2 poles (5.3051, 10.1158) (5.5154, 10.1158) (5.7524, 9.8934) (5.7524, 9.7037) knots 0 0 0 1 2 2 2
  spline S121 degree 2 poles (5.7524, 9.7037) (5.7524, 9.615) (5.7111, 9.4667) (5.6746, 9.4035) knots 0 0 0 1 2 2 2
  spline S122 degree 2 poles (5.6746, 9.4035) (5.6382, 9.3378) (5.5324, 9.209) (5.4741, 9.147) knots 0 0 0 1 2 2 2
  spline S123 degree 2 poles (5.4741, 9.147) (5.3793, 9.0437) (5.1471, 8.8224) (5.0778, 8.758) knots 0 0 0 1 2 2 2
  line L274 (5.0778, 8.758) -> (5.8144, 8.758)
  line L275 (5.8144, 8.758) -> (5.8144, 8.5842)
  spline S124 degree 2 poles (12.5378, 11.0733) (12.392, 11.0733) (12.1452, 11.1717) (12.0553, 11.2702) knots 0 0 0 1 2 2 2
  spline S125 degree 2 poles (12.0553, 11.2702) (11.9653, 11.3674) (11.8669, 11.6592) (11.8669, 11.8488) knots 0 0 0 1 2 2 2
  spline S126 degree 2 poles (11.8669, 11.8488) (11.8669, 12.0372) (11.9629, 12.3168) (12.0541, 12.4201) knots 0 0 0 1 2 2 2
  spline S127 degree 2 poles (12.0541, 12.4201) (12.144, 12.521) (12.3895, 12.6267) (12.5415, 12.6267) knots 0 0 0 1 2 2 2
  spline S128 degree 2 poles (12.5415, 12.6267) (12.6169, 12.6267) (12.7494, 12.6049) (12.8053, 12.5878) knots 0 0 0 1 2 2 2
  spline S129 degree 2 poles (12.8053, 12.5878) (12.8539, 12.572) (12.9548, 12.5271) (13.0046, 12.5003) knots 0 0 0 1 2 2 2
  line L276 (13.0046, 12.5003) -> (13.0046, 12.2596)
  line L277 (13.0046, 12.2596) -> (12.9888, 12.2596)
  spline S130 degree 2 poles (12.9888, 12.2596) (12.9621, 12.284) (12.8794, 12.352) (12.8199, 12.3848) knots 0 0 0 1 2 2 2
  spline S131 degree 2 poles (12.8199, 12.3848) (12.7627, 12.4165) (12.6278, 12.4566) (12.5403, 12.4566) knots 0 0 0 1 2 2 2
  spline S132 degree 2 poles (12.5403, 12.4566) (12.4442, 12.4566) (12.2729, 12.3776) (12.2084, 12.3022) knots 0 0 0 1 2 2 2
  spline S133 degree 2 poles (12.2084, 12.3022) (12.1452, 12.2256) (12.0747, 11.9934) (12.0747, 11.8488) knots 0 0 0 1 2 2 2
  spline S134 degree 2 poles (12.0747, 11.8488) (12.0747, 11.6944) (12.1489, 11.472) (12.2133, 11.3954) knots 0 0 0 1 2 2 2
  spline S135 degree 2 poles (12.2133, 11.3954) (12.2765, 11.3212) (12.4455, 11.2459) (12.5403, 11.2459) knots 0 0 0 1 2 2 2
  spline S136 degree 2 poles (12.5403, 11.2459) (12.6266, 11.2459) (12.7737, 11.2884) (12.8308, 11.32) knots 0 0 0 1 2 2 2
  spline S137 degree 2 poles (12.8308, 11.32) (12.8855, 11.3516) (12.9669, 11.4173) (12.99, 11.4404) knots 0 0 0 1 2 2 2
  line L278 (12.99, 11.4404) -> (13.0046, 11.4404)
  line L279 (13.0046, 11.4404) -> (13.0046, 11.2021)
  spline S138 degree 2 poles (13.0046, 11.2021) (12.9548, 11.179) (12.8673, 11.1365) (12.8053, 11.117) knots 0 0 0 1 2 2 2
  spline S139 degree 2 poles (12.8053, 11.117) (12.7396, 11.0951) (12.6278, 11.0733) (12.5378, 11.0733) knots 0 0 0 1 2 2 2
  line L280 (13.9977, 11.1) -> (13.266, 11.1)
  line L281 (13.266, 11.1) -> (13.266, 11.2532)
  line L282 (13.266, 11.2532) -> (13.5382, 11.2532)
  line L283 (13.5382, 11.2532) -> (13.5382, 12.2584)
  line L284 (13.5382, 12.2584) -> (13.266, 12.2584)
  line L285 (13.266, 12.2584) -> (13.266, 12.3958)
  spline S140 degree 2 poles (13.266, 12.3958) (13.4203, 12.3958) (13.5662, 12.4833) (13.5759, 12.6049) knots 0 0 0 1 2 2 2
  line L286 (13.5759, 12.6049) -> (13.7315, 12.6049)
  line L287 (13.7315, 12.6049) -> (13.7315, 11.2532)
  line L288 (13.7315, 11.2532) -> (13.9977, 11.2532)
  line L289 (13.9977, 11.2532) -> (13.9977, 11.1)
  spline S141 degree 2 poles (11.3134, 16.4799) (11.2696, 16.4692) (11.1743, 16.4575) (11.1267, 16.4575) knots 0 0 0 1 2 2 2
  spline S142 degree 2 poles (11.1267, 16.4575) (10.9915, 16.4575) (10.8233, 16.6083) (10.8155, 16.7483) knots 0 0 0 1 2 2 2
  spline S143 degree 2 poles (10.8155, 16.7483) (10.8048, 16.7483) (10.7863, 16.7483) (10.7786, 16.7483) knots 0 0 0 1 2 2 2
  spline S144 degree 2 poles (10.7786, 16.7483) (10.657, 16.7483) (10.4615, 16.831) (10.3915, 16.9117) knots 0 0 0 1 2 2 2
  spline S145 degree 2 poles (10.3915, 16.9117) (10.3225, 16.9914) (10.2486, 17.2248) (10.2486, 17.3726) knots 0 0 0 1 2 2 2
  spline S146 degree 2 poles (10.2486, 17.3726) (10.2486, 17.5243) (10.3235, 17.7538) (10.3925, 17.8355) knots 0 0 0 1 2 2 2
  spline S147 degree 2 poles (10.3925, 17.8355) (10.4625, 17.9162) (10.658, 17.9989) (10.7786, 17.9989) knots 0 0 0 1 2 2 2
  spline S148 degree 2 poles (10.7786, 17.9989) (10.9011, 17.9989) (11.0975, 17.9133) (11.1656, 17.8355) knots 0 0 0 1 2 2 2
  spline S149 degree 2 poles (11.1656, 17.8355) (11.2337, 17.7567) (11.3095, 17.5224) (11.3095, 17.3726) knots 0 0 0 1 2 2 2
  spline S150 degree 2 poles (11.3095, 17.3726) (11.3095, 17.1392) (11.1277, 16.8358) (10.9692, 16.7823) knots 0 0 0 1 2 2 2
  spline S151 degree 2 poles (10.9692, 16.7823) (10.973, 16.7376) (10.9964, 16.6656) (11.0149, 16.6452) knots 0 0 0 1 2 2 2
  spline S152 degree 2 poles (11.0149, 16.6452) (11.0372, 16.6199) (11.0985, 16.5966) (11.1529, 16.5966) knots 0 0 0 1 2 2 2
  spline S153 degree 2 poles (11.1529, 16.5966) (11.185, 16.5966) (11.2726, 16.617) (11.292, 16.6248) knots 0 0 0 1 2 2 2
  line L290 (11.292, 16.6248) -> (11.3134, 16.6248)
  line L291 (11.3134, 16.6248) -> (11.3134, 16.4799)
  spline S154 degree 2 poles (11.1432, 17.3726) (11.1432, 17.4922) (11.0917, 17.676) (11.045, 17.7363) knots 0 0 0 1 2 2 2
  spline S155 degree 2 poles (11.045, 17.7363) (10.9974, 17.7985) (10.8632, 17.8608) (10.7795, 17.8608) knots 0 0 0 1 2 2 2
  spline S156 degree 2 poles (10.7795, 17.8608) (10.693, 17.8608) (10.5627, 17.8005) (10.5131, 17.7363) knots 0 0 0 1 2 2 2
  spline S157 degree 2 poles (10.5131, 17.7363) (10.4654, 17.675) (10.4149, 17.4893) (10.4149, 17.3726) knots 0 0 0 1 2 2 2
  spline S158 degree 2 poles (10.4149, 17.3726) (10.4149, 17.1363) (10.6132, 16.8844) (10.7795, 16.8844) knots 0 0 0 1 2 2 2
  spline S159 degree 2 poles (10.7795, 16.8844) (10.9458, 16.8844) (11.1432, 17.1363) (11.1432, 17.3726) knots 0 0 0 1 2 2 2
  line L292 (12.1303, 16.7736) -> (11.5448, 16.7736)
  line L293 (11.5448, 16.7736) -> (11.5448, 16.8961)
  line L294 (11.5448, 16.8961) -> (11.7627, 16.8961)
  line L295 (11.7627, 16.8961) -> (11.7627, 17.7003)
  line L296 (11.7627, 17.7003) -> (11.5448, 17.7003)
  line L297 (11.5448, 17.7003) -> (11.5448, 17.8102)
  spline S160 degree 2 poles (11.5448, 17.8102) (11.6683, 17.8102) (11.785, 17.8802) (11.7928, 17.9775) knots 0 0 0 1 2 2 2
  line L298 (11.7928, 17.9775) -> (11.9173, 17.9775)
  line L299 (11.9173, 17.9775) -> (11.9173, 16.8961)
  line L300 (11.9173, 16.8961) -> (12.1303, 16.8961)
  line L301 (12.1303, 16.8961) -> (12.1303, 16.7736)
  point P0 (0, 0)
  point P1 (-6.4, 10.95)
  point P2 (-6.4, 7.75)
  point P3 (-6.4, 4.55)
  point P4 (0.6, 9.35)
  point P5 (0.6, 6.15)
  point P6 (0.6, 10.75)
  point P7 (8.9, 11.85)
  point P8 (-9.3, 10.95)
  point P9 (-6.4, 10.95)
  point P10 (3.2, 9.35)
  point P11 (3.5, 9.35)
  point P12 (0.6, 9.35)
  point P13 (0.6, 6.15)
  point P14 (8.9, 11.85)
  point P15 (8.05, 15.25)
  point P16 (-0.7, 14.5715)
  point P17 (-0.7, 14.5715)
  dimension "d0" = 34
  dimension "d1" = 55.5
  dimension "d16" = 2.8
  dimension "d17" = 5.2
  dimension "d18" = 15.4
  dimension "d19" = 8
  dimension "d22" = 3.2
  dimension "d27" = 15
  dimension "d28" = 17
  dimension "d30" = 3.2
  dimension "d31" = 5.5
  dimension "d32" = 14.5
  dimension "d33" = 0.3
  dimension "d46" = 0.3
  dimension "d55" = 1
  dimension "d56" = 3.5
  dimension "d57" = 2
  dimension "d62" = 1
  dimension "d63" = 2.5
  dimension "d64" = 3.8215
  dimension "d65" = 0.8
  dimension "d70" = 0.15
  dimension "d71" = 0.15
  dimension "d72" = 0.15
  dimension "d73" = 0.15
  dimension "d75" = 0.15
  dimension "d76" = 0.15
  dimension "d77" = 0.15
  dimension "d78" = 0.15
  constraints: 160 end point, 24 parallel, 23 midpoint, 12 perpendicular, 6 equal length, 6 horizontal, 3 collinear, 2 horizontal alignment, 1 vertical, 63 other
  measures "d16" distance of L2.end L0.start
  measures "d17" distance of L0.start L0.end
  measures "d18" distance between parallel lines of L6 L0
  measures "d19" distance between parallel lines of L7 L3
  measures "d22" distance of L0.start L8.start
  measures "d27" distance between parallel lines of L7 L23
  measures "d28" distance between parallel lines of L6 L22
  measures "d30" distance from line of L26 point (0.6, 10.75)
  measures "d31" distance between parallel lines of L38 L33
  measures "d32" distance between parallel lines of L6 L32
  measures "d33" distance from line of L3 point (-9.3, 10.95)
  measures "d46" distance of point (3.2, 9.35) point (3.5, 9.35)
  measures "d55" distance between parallel lines of L32 L65
  measures "d56" distance of L63.start L63.end
  measures "d57" distance of L65.end L63.start
  measures "d62" distance of L73.start L73.end
  measures "d63" distance of L73.end L74.end
  measures "d64" distance from line of L22 point (-0.7, 14.571)
  measures "d65" distance between parallel lines of L23 L76
  measures "d70" distance between parallel lines of L0 L87
  measures "d71" distance between parallel lines of L8 L91
  measures "d72" distance between parallel lines of L95 L14
  measures "d73" distance between parallel lines of L28 L105
  measures "d75" distance between parallel lines of L22 L99
  measures "d76" distance between parallel lines of L32 L107
  measures "d77" distance between parallel lines of L63 L111
  measures "d78" distance between parallel lines of L73 L115
emboss "Sbalzo1" sketch "Schizzo4" operation add depth 0.05 direction (0, 0, -1)
sketch "Schizzo5" plane through (0, 0, 0.55) normal (0, 0, 1) x (1, 0, 0)
  line L0 (-2.5, 25.25) -> (0, 25.25)
  line L1 (0, 25.25) -> (0, 27.75)
  line L2 (0, 27.75) -> (-2.5, 27.75)
  line L3 (-2.5, 27.75) -> (-2.5, 25.25)
  line L4 (-2.5, 25.25) -> (0, 27.75) construction
  line L5 (0, 25.25) -> (-2.5, 27.75) construction
  line L6 (15, 27.75) -> (-15, 27.75) construction
  point P0 (0, 0)
  point P1 (-1.25, 26.5)
  point P2 (0, 26.5)
  dimension "d81" = 2.5
  constraints: 12 end point, 3 midpoint, 2 parallel, 2 perpendicular, 1 collinear, 1 horizontal, 1 vertical alignment
  measures "d81" distance between parallel lines of L1 L3
extrude "Estrusione3" add sketch "Schizzo5" along normal blind 2.6 separate body
sketch "Schizzo6" plane through (0, 0, 3.15) normal (0, 0, 1) x (1, 0, 0)
  line L0 (-1.5, 26.25) -> (-1, 26.25)
  line L1 (-1, 26.25) -> (-1, 26.75)
  line L2 (-1, 26.75) -> (-1.5, 26.75)
  line L3 (-1.5, 26.75) -> (-1.5, 26.25)
  line L4 (-1.5, 26.25) -> (-1, 26.75) construction
  line L5 (-1, 26.25) -> (-1.5, 26.75) construction
  line L6 (-2.5, 25.25) -> (0, 25.25) construction
  line L7 (-2.5, 27.75) -> (-2.5, 25.25) construction
  point P0 (0, 0)
  point P1 (-1.25, 26.5)
  point P2 (-1.25, 25.25)
  point P3 (-2.5, 26.5)
  dimension "d84" = 0.5
  constraints: 12 end point, 4 midpoint, 2 parallel, 2 perpendicular, 1 horizontal, 1 horizontal alignment, 1 vertical alignment
  measures "d84" distance of L0.start L0.end
extrude "Estrusione4" add sketch "Schizzo6" along normal blind 5.5 and the other way blind 5.5 separate body
chamfer "Smusso1" distance 0.15 angle 45 8 edges at (-1, 26.5, 8.65) (-1.25, 26.75, 8.65) (-1.5, 26.5, 8.65) (-1.25, 26.25, 8.65) (-1.25, 26.75, -2.35) (-1, 26.5, -2.35) (-1.5, 26.5, -2.35) (-1.25, 26.25, -2.35)
chamfer "Smusso2" distance 0.5 angle 45 4 edges at (0, 25.25, 1.85) (0, 27.75, 1.85) (-2.5, 27.75, 1.85) (-2.5, 25.25, 1.85)
pattern_linear "Serie rettangolare1" count 8 spacing 2.5 along (1, 0, 0) first direction both ways yes bodies 2 3
sketch "Schizzo7" plane through (0, 0, 0.55) normal (0, 0, 1) x (1, 0, 0)
  circle A0 centre (-6.25, 24.05) radius 1
  line L0 (-7, 25.25) -> (-5.5, 25.25) construction
  point P0 (0, 0)
  point P1 (-6.25, 25.25)
  dimension "d96" = 2
  dimension "d97" = 1.2
  constraints: 1 centre point, 1 midpoint, 1 vertical alignment
  measures "d96" diameter of A0
  measures "d97" distance from line of L0 A0.centre
extrude "Estrusione5" add sketch "Schizzo7" along normal blind 0.05 bodies 1
mirror "Specchio2" about plane through (0, 0, 0) normal (0, 0, 1) of "Estrusione5" bodies 1
sketch "Schizzo8" plane through (-6.25, 24.05, 0.6) normal (0, 0, 1) x (1, 0, 0)
  circle A0 centre (0, 0) radius 1 construction
  point P0 (6.25, -24.05)
  constraints: 1 coincident
hole "Foro2" at (-6.25, 24.05, 0.6) direction (0, 0, -1) diameter 1 end through all bodies 1
pattern_linear "Serie rettangolare2" count 6 spacing 2.5 along (1, 0, 0) of "Estrusione5", "Specchio2", "Foro2" bodies 1
sketch "Schizzo9" plane through (0, 0, -0.55) normal (0, 0, -1) x (-1, 0, 0)
  line L0 (17, 25.75) -> (17, -25.75) construction
  line L1 (-17, -25.75) -> (-17, 25.75) construction
  line L2 (17, 22.55) -> (-17, 22.55)
  line L3 (-17, 22.55) -> (-17, -21.15)
  line L4 (-17, -21.15) -> (17, -21.15)
  line L5 (17, -21.15) -> (17, 22.55)
  line L6 (15, 27.75) -> (-15, 27.75) construction
  line L7 (16.5, 22.05) -> (-16.5, 22.05)
  line L8 (-16.5, 22.05) -> (-16.5, -19.65)
  line L9 (-16.5, -19.65) -> (16.5, -19.65)
  line L10 (16.5, -19.65) -> (16.5, 22.05)
  point P0 (0, 0)
  dimension "d112" = 5.2
  dimension "d113" = 43.7
  dimension "d114" = 0.5
  dimension "d115" = 0.5
  dimension "d116" = 0.5
  dimension "d117" = 1.5
  constraints: 16 end point, 4 parallel, 2 horizontal, 2 perpendicular, 2 point on line
  measures "d112" distance between parallel lines of L6 L2
  measures "d113" distance between parallel lines of L4 L2
  measures "d114" distance between parallel lines of L0 L10
  measures "d115" distance between parallel lines of L2 L7
  measures "d116" distance between parallel lines of L1 L8
  measures "d117" distance between parallel lines of L4 L9
extrude "Estrusione6" add sketch "Schizzo9" along normal blind 3.1 separate body
sketch "Schizzo10" plane through (0, 0, -3.65) normal (0, 0, -1) x (-1, 0, 0)
  line L0 (16.5, -19.65) -> (-16.5, -19.65) construction
  line L1 (-17, -21.15) -> (17, -21.15) construction
  line L2 (14, -19.65) -> (-14, -19.65)
  line L3 (-14, -19.65) -> (-14, -21.15)
  line L4 (-14, -21.15) -> (14, -21.15)
  line L5 (14, -21.15) -> (14, -19.65)
  line L6 (17, -21.15) -> (17, 22.55) construction
  line L7 (-17, 22.55) -> (-17, -21.15) construction
  point P0 (0, 0)
  dimension "d120" = 3
  dimension "d121" = 3
  constraints: 8 end point, 2 parallel, 2 point on line, 1 horizontal, 1 perpendicular
  measures "d120" distance between parallel lines of L5 L6
  measures "d121" distance between parallel lines of L7 L3
extrude "Estrusione7" cut sketch "Schizzo10" against normal blind 2.5 bodies 4
sketch "Schizzo11" plane through (0, 0, -0.55) normal (0, 0, -1) x (-1, 0, 0)
  line L0 (16.5, 22.05) -> (16.5, -19.65) construction
  line L1 (-16.5, 22.05) -> (16.5, 22.05) construction
  line L2 (-16.5, -19.65) -> (-16.5, 22.05) construction
  line L3 (-14, -19.65) -> (14, -19.65) construction
  line L4 (16.5, -19.65) -> (14, -19.65) construction
  line L5 (-14, -19.65) -> (-16.5, -19.65) construction
  line L6 (16.3, 21.85) -> (-16.3, 21.85)
  line L7 (-16.3, 21.85) -> (-16.3, -19.45)
  line L8 (-16.3, -19.45) -> (16.3, -19.45)
  line L9 (16.3, -19.45) -> (16.3, 21.85)
  point P0 (0, 0)
  point P1 (15.25, -19.65)
  dimension "d124" = 0.2
  dimension "d125" = 0.2
  dimension "d126" = 0.2
  dimension "d127" = 0.2
  constraints: 8 end point, 2 parallel, 1 horizontal, 1 midpoint, 1 perpendicular
  measures "d124" distance between parallel lines of L0 L9
  measures "d125" distance between parallel lines of L1 L6
  measures "d126" distance between parallel lines of L2 L7
  measures "d127" distance from line of point (15.25, -19.65) L8
extrude "Estrusione8" add sketch "Schizzo11" along normal up to surface (3.1 mm away) separate body
sketch "Schizzo12" plane through (0, 0, 0) normal (1, 0, 0) x (0, 1, 0)
  line L0 (27.75, -0.55) -> (-27.75, -0.55) construction
  line L1 (-27.75, -0.55) -> (-27.75, 0.55) construction
  line L2 (-27.75, 0.55) -> (4.75, 0.55) construction
  line L3 (4.75, 0.55) -> (4.75, 0.6) construction
  line L4 (4.75, 0.6) -> (4.9, 0.6) construction
  line L5 (4.9, 0.6) -> (4.9, 0.55) construction
  line L6 (4.9, 0.55) -> (7.4, 0.55) construction
  line L7 (7.4, 0.55) -> (7.4, 0.6) construction
  line L8 (7.4, 0.6) -> (7.55, 0.6) construction
  line L9 (7.55, 0.6) -> (7.55, 0.55) construction
  line L10 (7.55, 0.55) -> (7.95, 0.55) construction
  line L11 (7.95, 0.55) -> (7.95, 0.6) construction
  line L12 (7.95, 0.6) -> (8.1, 0.6) construction
  line L13 (8.1, 0.6) -> (8.1, 0.55) construction
  line L14 (8.1, 0.55) -> (10.6, 0.55) construction
  line L15 (10.6, 0.55) -> (10.6, 0.6) construction
  line L16 (10.6, 0.6) -> (10.75, 0.6) construction
  line L17 (10.75, 0.6) -> (10.75, 0.55) construction
  line L18 (10.75, 0.55) -> (27.75, 0.55) construction
  line L19 (27.75, 0.55) -> (27.75, -0.55) construction
  line L20 (27.25, 3.15) -> (27.25, 0.55) construction
  line L21 (27.25, 0.55) -> (25.75, 0.55) construction
  line L22 (25.75, 0.55) -> (25.75, 3.15) construction
  line L23 (25.75, 3.15) -> (27.25, 3.15) construction
  line L24 (-19.65, -1.15) -> (-21.15, -1.15) construction
  line L25 (-21.15, -1.15) -> (-21.15, -0.55) construction
  line L26 (-21.15, -0.55) -> (-19.65, -0.55) construction
  line L27 (-19.65, -0.55) -> (-19.65, -1.15) construction
  line L28 (22.55, -3.65) -> (22.05, -3.65) construction
  line L29 (22.05, -3.65) -> (22.05, -0.55) construction
  line L30 (22.05, -0.55) -> (22.55, -0.55) construction
  line L31 (22.55, -0.55) -> (22.55, -3.65) construction
  line L32 (21.85, -0.55) -> (21.85, -3.65) construction
  line L33 (21.85, -3.65) -> (-19.45, -3.65) construction
  line L34 (-19.45, -3.65) -> (-19.45, -0.55) construction
  line L35 (-19.45, -0.55) -> (21.85, -0.55) construction
  arc A0 (-21.15, -0.55) -> (-21.15, -2.55) centre (-21.15, -1.55) ccw
  line L36 (-21.15, -2.55) -> (-19.45, -2.55)
  line L37 (-19.45, -2.45) -> (-21.15, -2.45)
  arc A1 (-21.15, -0.65) -> (-21.15, -2.45) centre (-21.15, -1.55) ccw
  line L38 (-19.45, -2.45) -> (-19.45, -2.55)
  line L39 (-21.15, -0.55) -> (-21.15, -0.65)
  point P0 (0, 0)
  dimension "d130" = 1
  dimension "d131" = 0.1
  constraints: 8 end point, 4 point on circle, 2 centre point, 2 tangent, 1 collinear, 1 horizontal, 1 parallel, 1 point on line, 1 other
  measures "d130" radius of A0
  measures "d131" distance between parallel lines of L36 L37
extrude "Estrusione9" add sketch "Schizzo12" along normal blind 8 and the other way blind 10 separate body